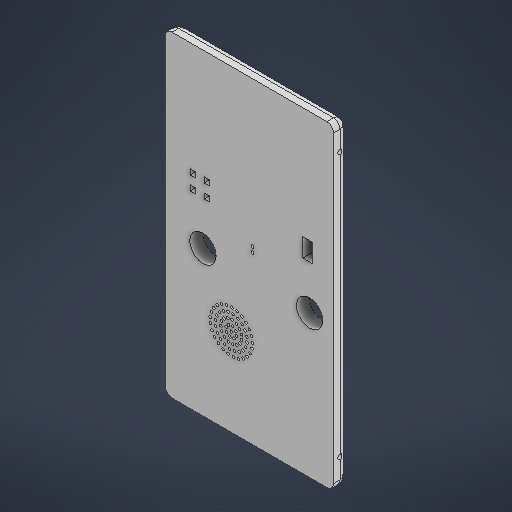
# Autodesk Inventor part: Top_Shell
Saved by Autodesk Inventor 2027 (Build 310192000, 192)
## iProperties
Created: 2026-03-03
Part Number: Top_Shell
Material: Generic
Document SubType Name: Modeling
Designer: kjedr
Density: 1 g/cm^3
Appearance: Default
Author: kjedr
Autodesk Inventor part; units mm, degrees
ref_plane "YZ Plane" through (0, 0, 0) normal (1, 0, 0) x (0, 1, 0)
ref_plane "XZ Plane" through (0, 0, 0) normal (0, 1, 0) x (-1, 0, 0)
ref_plane "XY Plane" through (0, 0, 0) normal (0, 0, 1) x (1, 0, 0)
sketch "Sketch1" plane through (0, 0, 0) normal (0, 0, 1) x (1, 0, 0)
  line L0 (0, 0) -> (80.8355, 0)
  line L1 (80.8355, 0) -> (80.8355, 152.4)
  line L2 (80.8355, 152.4) -> (0, 152.4)
  line L3 (0, 152.4) -> (0, 0)
  dimension "d0" = 80.8355
  dimension "d1" = 152.4
  constraints: 8 end point, 3 perpendicular, 1 horizontal
  measures "d0" distance of L2.end L1.end
  measures "d1" distance of L1.end L0.end
extrude "Extrusion1" add sketch "Sketch1" along normal blind 6.35
fillet "Fillet1" radius 3.175 8 edges at (80.8355, 152.4, 3.175) (0, 152.4, 3.175) (40.4178, 152.4, 0) (80.8355, 76.2, 0) (40.4177, 0, 0) (0, 76.2, 0) (0, 0, 3.175) (80.8355, 0, 3.175)
sketch "Sketch8" plane through (0, 0, 0) normal (0, 0, -1) x (-1, 0, 0)
  circle A0 centre (-31.7043, 41.9898) radius 12.7 construction
  circle A1 centre (-31.7043, 41.9898) radius 10.16 construction
  circle A2 centre (-31.7043, 41.9898) radius 7.62 construction
  circle A3 centre (-31.7043, 41.9898) radius 5.08 construction
  circle A4 centre (-31.7043, 41.9898) radius 2.54 construction
  line L0 (-80.8355, 149.225) -> (-80.8355, 3.175) projected
  line L1 (-77.6605, 0) -> (-3.175, 0) projected
  point P0 (0, 0)
  point P1 (-29.2552, 42.6633)
  point P2 (-36.6993, 41.0645)
  point P3 (-24.1328, 42.8482)
  point P4 (-22.1292, 45.3874)
  point P5 (-23.275, 47.6618)
  point P6 (-24.9504, 49.5799)
  point P7 (-27.0501, 51.0211)
  point P8 (-29.4424, 51.8948)
  point P9 (-31.9767, 52.1461)
  point P10 (-34.4939, 51.7593)
  point P11 (-36.8359, 50.7586)
  point P12 (-38.8554, 49.2069)
  point P13 (-40.4255, 47.2018)
  point P14 (-41.4477, 44.8691)
  point P15 (-41.8577, 42.3556)
  point P16 (-41.6297, 39.819)
  point P17 (-40.778, 37.4189)
  point P18 (-39.3562, 35.3059)
  point P19 (-37.4536, 33.613)
  point P20 (-35.1898, 32.4463)
  point P21 (-32.7069, 31.8794)
  point P22 (-30.161, 31.9477)
  point P23 (-27.7122, 32.6469)
  point P24 (-25.5141, 33.9332)
  point P25 (-23.705, 35.7258)
  point P26 (-22.3985, 37.9119)
  point P27 (-21.6768, 40.3543)
  point P28 (-21.5851, 42.8994)
  point P29 (-24.7686, 45.1459)
  point P30 (-26.0834, 47.1347)
  point P31 (-27.9483, 48.6198)
  point P32 (-30.1809, 49.4559)
  point P33 (-32.5627, 49.5613)
  point P34 (-34.8604, 48.9254)
  point P35 (-36.8492, 47.6107)
  point P36 (-38.3343, 45.7457)
  point P37 (-39.1704, 43.5131)
  point P38 (-39.2758, 41.1313)
  point P39 (-38.6399, 38.8336)
  point P40 (-37.3252, 36.8449)
  point P41 (-35.4602, 35.3597)
  point P42 (-33.2276, 34.5236)
  point P43 (-30.8458, 34.4183)
  point P44 (-28.5481, 35.0541)
  point P45 (-26.5594, 36.3689)
  point P46 (-25.0742, 38.2338)
  point P47 (-24.2381, 40.4664)
  point P48 (-35.8911, 39.1129)
  point P49 (-34.359, 37.6586)
  point P50 (-32.3679, 36.9533)
  point P51 (-30.262, 37.1188)
  point P52 (-28.4055, 38.1266)
  point P53 (-27.1194, 39.8023)
  point P54 (-26.626, 41.8562)
  point P55 (-27.0107, 43.9333)
  point P56 (-28.207, 45.6743)
  point P57 (-30.008, 46.7782)
  point P58 (-32.1023, 47.0541)
  point P59 (-34.1278, 46.4544)
  point P60 (-35.7342, 45.0827)
  point P61 (-36.6438, 43.1762)
  point P62 (-30.4487, 44.1978)
  point P63 (-32.3778, 44.4388)
  point P64 (-33.9123, 43.2453)
  point P65 (-34.1533, 41.3163)
  point P66 (-32.9598, 39.7818)
  point P67 (-31.0308, 39.5407)
  point P68 (-29.4963, 40.7343)
  dimension "d39" = 20.32
  dimension "d40" = 15.24
  dimension "d41" = 10.16
  dimension "d42" = 5.08
  dimension "d38" = 25.4
  dimension "d45" = 360
  dimension "d49" = 360
  dimension "d53" = 360
  dimension "d57" = 360
  constraints: 5 coincident, 1 centre point, 84 other
  measures "d38" diameter of A0
hole "Hole1" at (31.7043, 41.9898, 0) at (29.2552, 42.6633, 0) at (36.6993, 41.0645, 0) at (24.1328, 42.8482, 0) at (22.1292, 45.3874, 0) at (23.275, 47.6618, 0) at (24.9504, 49.5799, 0) at (27.0501, 51.0211, 0) at (29.4424, 51.8948, 0) at (31.9767, 52.1461, 0) at (34.4939, 51.7593, 0) at (36.8359, 50.7586, 0) at (38.8554, 49.2069, 0) at (40.4255, 47.2018, 0) at (41.4477, 44.8691, 0) at (41.8577, 42.3556, 0) at (41.6297, 39.819, 0) at (40.778, 37.4189, 0) at (39.3562, 35.3059, 0) at (37.4536, 33.613, 0) at (35.1898, 32.4463, 0) at (32.7069, 31.8794, 0) at (30.161, 31.9477, 0) at (27.7122, 32.6469, 0) at (25.5141, 33.9332, 0) at (23.705, 35.7258, 0) at (22.3985, 37.9119, 0) at (21.6768, 40.3543, 0) at (21.5851, 42.8994, 0) at (24.7686, 45.1459, 0) at (26.0834, 47.1347, 0) at (27.9483, 48.6198, 0) at (30.1809, 49.4559, 0) at (32.5627, 49.5613, 0) at (34.8604, 48.9254, 0) at (36.8492, 47.6107, 0) at (38.3343, 45.7457, 0) at (39.1704, 43.5131, 0) at (39.2758, 41.1313, 0) at (38.6399, 38.8336, 0) at (37.3252, 36.8449, 0) at (35.4602, 35.3597, 0) at (33.2276, 34.5236, 0) at (30.8458, 34.4183, 0) at (28.5481, 35.0541, 0) at (26.5594, 36.3689, 0) at (25.0742, 38.2338, 0) at (24.2381, 40.4664, 0) at (35.8911, 39.1129, 0) at (34.359, 37.6586, 0) direction (0, 0, 1) diameter 1.27 end through all and at (32.3679, 36.9533, 0) (30.262, 37.1188, 0) (28.4055, 38.1266, 0) (27.1194, 39.8023, 0) (26.626, 41.8562, 0) (27.0107, 43.9333, 0) (28.207, 45.6743, 0) (30.008, 46.7782, 0) (32.1023, 47.0541, 0) (34.1278, 46.4544, 0) (35.7342, 45.0827, 0) (36.6438, 43.1762, 0) (30.4487, 44.1978, 0) (32.3778, 44.4388, 0) (33.9123, 43.2453, 0) (34.1533, 41.3163, 0) (32.9598, 39.7818, 0) (31.0308, 39.5407, 0) (29.4963, 40.7343, 0)
sketch "Sketch12" plane through (0, 0, 0) normal (0, 0, -1) x (-1, 0, 0)
  point P0 (0, 0)
sketch "Sketch14" plane through (0, 0, 0) normal (0, 0, -1) x (-1, 0, 0)
  line L0 (-75.6868, 90.81) -> (-5.1488, 90.81) construction
  line L1 (-5.1488, 90.81) -> (-5.1488, 6.81) construction
  line L2 (-5.1488, 6.81) -> (-75.6868, 6.81) construction
  line L3 (-75.6868, 6.81) -> (-75.6868, 90.81) construction
  circle A0 centre (-75.2472, 83.516) radius 1.6
  circle A1 centre (-13.6268, 83.516) radius 1.6
  circle A2 centre (-75.2472, 22.81) radius 1.6
  circle A3 centre (-13.6268, 22.81) radius 1.6
  line L4 (-77.6605, 149.225) -> (-3.175, 149.225) projected
  line L5 (-77.0255, 3.81) -> (-3.81, 3.81) projected
  point P0 (0, 0)
  point P1 (-40.4178, 90.81)
  point P2 (-40.4178, 125.7733)
  point P3 (-69.4004, 68.5651)
  point P4 (-18.0721, 69.8455)
  point P5 (-40.4178, 6.81)
  point P6 (-40.4178, 149.225)
  dimension "d90" = 3.2
  constraints: 8 end point, 4 centre point, 4 vertical alignment, 3 equal radius, 3 midpoint, 2 horizontal alignment, 2 parallel, 1 horizontal, 1 perpendicular
  measures "d90" diameter of A0
hole "Hole4" at (69.4004, 68.5651, 0) at (18.0721, 69.8455, 0) direction (0, 0, 1) diameter 12.7 end through all
sketch "Sketch22" plane through (0, 3.175, 3.175) normal (-1, 0, 0) x (0, 0, 1)
  line L0 (3.175, 146.05) -> (3.175, 0) projected
  line L1 (0, -3.175) -> (3.175, -3.175) projected
  line L2 (3.175, 149.225) -> (0, 149.225) projected
  point P0 (-3.175, -3.175)
  point P1 (0, 9.525)
  point P2 (0, 136.525)
  dimension "d158" = 3.175
  dimension "d159" = 12.7
  dimension "d160" = 3.175
  dimension "d161" = 12.7
  measures "d158" distance from line of L0 point (0, 9.525)
  measures "d159" distance from line of L1 point (0, 9.525)
  measures "d160" distance from line of L0 point (0, 136.525)
  measures "d161" distance from line of L2 point (0, 136.525)
sketch "Sketch23" plane through (80.8355, 3.175, 6.35) normal (1, 0, 0) x (0, 0, -1)
  line L0 (0, 0) -> (0, 146.05) projected
  line L1 (3.175, 149.225) -> (0, 149.225) projected
  line L2 (0, -3.175) -> (3.175, -3.175) projected
  point P0 (6.35, -3.175)
  point P1 (3.175, 9.525)
  point P2 (3.175, 136.525)
  point P3 (1.5875, 149.225)
  dimension "d162" = 3.175
  dimension "d163" = 12.7
  dimension "d164" = 12.7
  dimension "d165" = 3.175
  constraints: 1 midpoint
  measures "d162" distance from line of L0 point (3.175, 136.525)
  measures "d163" vertical distance of point (1.587, 149.225) point (3.175, 136.525)
  measures "d164" distance from line of L2 point (3.175, 9.525)
  measures "d165" distance from line of L0 point (3.175, 9.525)
hole "Hole6" at (80.8355, 139.7, 3.175) at (80.8355, 12.7, 3.175) direction (-1, 0, 0) diameter 2.286 depth 25.4
hole "Hole7" at (0, 12.7, 3.175) at (0, 139.7, 3.175) direction (1, 0, 0) diameter 2.286 depth 25.4
sketch "Sketch24" plane through (0, 0, 0) normal (0, 0, -1) x (-1, 0, 0)
  line L0 (-19.86, 98.6) -> (-13.16, 98.6)
  line L1 (-13.16, 98.6) -> (-13.16, 91.9)
  line L2 (-13.16, 91.9) -> (-19.86, 91.9)
  line L3 (-19.86, 91.9) -> (-19.86, 98.6)
  line L4 (0, 13.843) -> (0, 138.557) projected
  line L5 (-3.175, 152.4) -> (-77.6605, 152.4) projected
  point P0 (0, 0)
  point P1 (-16.51, 98.6)
  point P2 (-13.16, 95.25)
  dimension "d200" = 6.7
  dimension "d201" = 6.7
  dimension "d202" = 16.51
  dimension "d203" = 57.15
  constraints: 8 end point, 2 midpoint, 2 parallel, 1 horizontal, 1 perpendicular
  measures "d200" distance of L1.end L2.end
  measures "d201" distance of L0.end L1.end
  measures "d202" distance from line of L4 point (-16.51, 98.6)
  measures "d203" distance from line of L5 point (-13.16, 95.25)
extrude "Extrusion15" cut sketch "Sketch24" against normal blind 3.5
sketch "Sketch25" plane through (0, 0, 0) normal (0, 0, -1) x (-1, 0, 0)
  line L0 (-21.13, 99.87) -> (-18.59, 99.87)
  line L1 (-18.59, 99.87) -> (-18.59, 97.33)
  line L2 (-18.59, 97.33) -> (-21.13, 97.33)
  line L3 (-21.13, 97.33) -> (-21.13, 99.87)
  line L4 (-19.86, 91.9) -> (-19.86, 98.6) projected
  line L5 (-21.13, 99.87) -> (-18.59, 97.33) construction
  line L6 (-18.59, 99.87) -> (-21.13, 97.33) construction
  line L7 (-14.43, 99.87) -> (-11.89, 99.87)
  line L8 (-11.89, 99.87) -> (-11.89, 97.33)
  line L9 (-11.89, 97.33) -> (-14.43, 97.33)
  line L10 (-14.43, 97.33) -> (-14.43, 99.87)
  line L11 (-19.86, 98.6) -> (-13.16, 98.6) projected
  line L12 (-14.43, 99.87) -> (-11.89, 97.33) construction
  line L13 (-11.89, 99.87) -> (-14.43, 97.33) construction
  line L14 (-14.43, 93.17) -> (-11.89, 93.17)
  line L15 (-11.89, 93.17) -> (-11.89, 90.63)
  line L16 (-11.89, 90.63) -> (-14.43, 90.63)
  line L17 (-14.43, 90.63) -> (-14.43, 93.17)
  line L18 (-13.16, 91.9) -> (-19.86, 91.9) projected
  line L19 (-14.43, 93.17) -> (-11.89, 90.63) construction
  line L20 (-11.89, 93.17) -> (-14.43, 90.63) construction
  line L21 (-21.13, 93.17) -> (-18.59, 93.17)
  line L22 (-18.59, 93.17) -> (-18.59, 90.63)
  line L23 (-18.59, 90.63) -> (-21.13, 90.63)
  line L24 (-21.13, 90.63) -> (-21.13, 93.17)
  line L25 (-21.13, 93.17) -> (-18.59, 90.63) construction
  line L26 (-18.59, 93.17) -> (-21.13, 90.63) construction
  point P0 (0, 0)
  point P1 (-18.59, 91.9)
  point P2 (-19.86, 93.17)
  dimension "d206" = 2.54
  dimension "d207" = 2.54
  dimension "d208" = 2.54
  dimension "d209" = 2.54
  dimension "d210" = 2.54
  dimension "d211" = 2.54
  dimension "d212" = 2.54
  dimension "d213" = 2.54
  constraints: 48 end point, 8 midpoint, 8 parallel, 4 horizontal, 4 perpendicular
  measures "d206" distance of L1.end L2.end
  measures "d207" distance of L0.end L1.end
  measures "d208" distance of L8.end L9.end
  measures "d209" distance of L7.end L8.end
  measures "d210" distance of L15.end L16.end
  measures "d211" distance of L14.end L15.end
  measures "d212" distance of L22.end L23.end
  measures "d213" distance of L21.end L22.end
extrude "Extrusion16" cut sketch "Sketch25" against normal up to next
sketch "Sketch26" plane through (0, 0, 6.35) normal (0, 0, 1) x (1, 0, 0)
  line L0 (66.1035, 98.679) -> (70.6755, 98.679)
  line L1 (70.6755, 98.679) -> (70.6755, 89.789)
  line L2 (70.6755, 89.789) -> (66.1035, 89.789)
  line L3 (66.1035, 89.789) -> (66.1035, 98.679)
  line L4 (66.1035, 98.679) -> (70.6755, 89.789) construction
  line L5 (70.6755, 98.679) -> (66.1035, 89.789) construction
  line L6 (80.8355, 3.175) -> (80.8355, 149.225) projected
  line L7 (77.6605, 152.4) -> (3.175, 152.4) projected
  line L8 (67.3481, 98.044) -> (69.4309, 98.044)
  line L9 (69.4309, 98.044) -> (69.4309, 90.424)
  line L10 (69.4309, 90.424) -> (67.3481, 90.424)
  line L11 (67.3481, 90.424) -> (67.3481, 98.044)
  line L12 (67.3481, 98.044) -> (69.4309, 90.424) construction
  line L13 (69.4309, 98.044) -> (67.3481, 90.424) construction
  point P0 (0, 0)
  point P1 (68.3895, 94.234)
  dimension "d216" = 4.572
  dimension "d217" = 8.89
  dimension "d218" = 10.16
  dimension "d219" = 53.721
  dimension "d220" = 2.0828
  dimension "d221" = 7.62
  constraints: 24 end point, 4 midpoint, 4 parallel, 2 horizontal, 2 perpendicular
  measures "d216" distance of L1.end L2.end
  measures "d217" distance of L0.end L1.end
  measures "d218" distance between parallel lines of L6 L1
  measures "d219" distance between parallel lines of L7 L0
  measures "d220" distance of L9.end L10.end
  measures "d221" distance of L8.end L9.end
extrude "Extrusion17" cut sketch "Sketch26" against normal up to next contours L8 L9 L10 L11
extrude "Extrusion18" cut sketch "Sketch26" against normal blind 5.842
sketch "Sketch27" plane through (0, 0, 0) normal (0, 0, -1) x (-1, 0, 0)
  circle A0 centre (-41.91, 81.28) radius 3
  line L0 (0, 13.843) -> (0, 138.557) projected
  line L1 (-77.6605, 0) -> (-3.175, 0) projected
  circle A1 centre (-41.91, 82.53) radius 0.6985
  circle A2 centre (-41.91, 80.03) radius 0.6985
  point P0 (0, 0)
  dimension "d226" = 6
  dimension "d227" = 41.91
  dimension "d228" = 81.28
  dimension "d229" = 1.397
  dimension "d230" = 1.397
  dimension "d231" = 2.5
  dimension "d232" = 1.25
  constraints: 3 centre point, 2 vertical alignment
  measures "d226" diameter of A0
  measures "d227" distance from line of L0 A0.centre
  measures "d228" distance from line of L1 A0.centre
  measures "d229" diameter of A1
  measures "d230" diameter of A2
  measures "d231" distance of A2.centre A1.centre
  measures "d232" distance of A0.centre A2.centre
extrude "Extrusion19" cut sketch "Sketch27" against normal through all contours A1 | A2
extrude "Extrusion20" cut sketch "Sketch27" against normal blind 1
body "Solid1"
